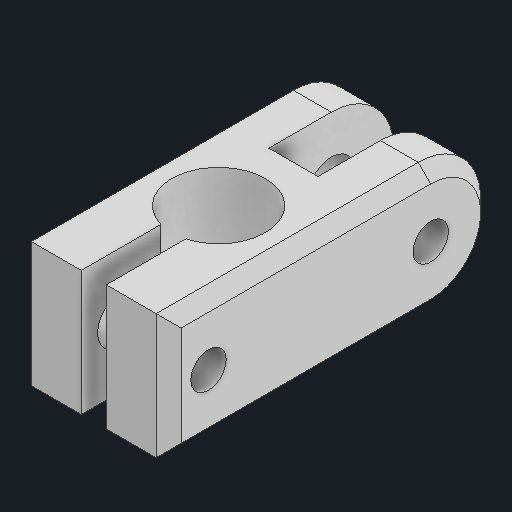
# Autodesk Inventor part: Part1
Saved by Autodesk Inventor 2025.1 (Build 291241020, 241B)
## iProperties
Created: 2025-05-01
Part Number: Part1
Material: Generic
Document SubType Name: Modeling
Designer: Joshua Eah
Density: 1 g/cm^3
Appearance: Default
Author: Joshua Eah
Autodesk Inventor part; units mm, degrees
ref_plane "YZ Plane" through (0, 0, 0) normal (1, 0, 0) x (0, 1, 0)
ref_plane "XZ Plane" through (0, 0, 0) normal (0, 1, 0) x (-1, 0, 0)
ref_plane "XY Plane" through (0, 0, 0) normal (0, 0, 1) x (1, 0, 0)
sketch "Sketch1" plane through (0, 0, 0) normal (0, 1, 0) x (-1, 0, 0)
  circle A0 centre (0, 0) radius 4.7625
  line L0 (7.62, -20.32) -> (-7.62, -20.32)
  line L1 (-7.62, -20.32) -> (-7.62, 12.7)
  line L2 (-7.62, 12.7) -> (7.62, 12.7)
  line L3 (7.62, 12.7) -> (7.62, -20.32)
  line L4 (1.27, 4.59) -> (1.27, 12.7)
  line L5 (-1.27, 4.59) -> (-1.27, 12.7)
  line L6 (0, 4.7625) -> (0, 12.7) construction
  dimension "d0" = 9.525
  dimension "d1" = 7.62
  dimension "d2" = 7.62
  dimension "d3" = 20.32
  dimension "d4" = 12.7
  dimension "d6" = 1.27
  dimension "d7" = 1.27
  constraints: 14 end point, 3 perpendicular, 3 point on circle, 2 parallel, 2 point on line, 1 centre point, 1 coincident, 1 horizontal, 1 midpoint
  measures "d0" diameter of A0
  measures "d1" distance from line of L3 A0.centre
  measures "d2" distance from line of L1 A0.centre
  measures "d3" distance from line of L0 A0.centre
  measures "d4" distance from line of L2 A0.centre
  measures "d6" distance between parallel lines of L4 L6
  measures "d7" distance between parallel lines of L5 L6
extrude "Extrusion1" add sketch "Sketch1" along normal blind 12.7 contours A0 L4 L2 L3 L0 L1 L5
sketch "Sketch2" plane through (-7.62, 0, -20.32) normal (-1, 0, 0) x (0, 0, 1)
  line L0 (0, 0) -> (33.02, 0) projected
  line L1 (33.02, 0) -> (33.02, 12.7) projected
  line L2 (0, 12.7) -> (33.02, 12.7) projected
  line L3 (0, 0) -> (0, 12.7) projected
  line L4 (0, 6.35) -> (33.02, 6.35) construction
  circle A0 centre (28.9687, 6.35) radius 1.75
  circle A1 centre (6.35, 6.35) radius 1.5
  point P0 (20.32, 0)
  dimension "d10" = 3.5
  dimension "d11" = 4.0513
  dimension "d20" = 3
  dimension "d21" = 6.35
  constraints: 2 centre point, 2 end point, 2 midpoint, 2 point on line
  measures "d10" diameter of A0
  measures "d11" distance from line of L1 A0.centre
  measures "d20" diameter of A1
  measures "d21" distance from line of A1.centre L3
hole "Hole1" at (-7.62, 6.35, 8.6487) at (-7.62, 6.35, -13.97) direction (1, 0, 0) diameter 3.6068 end through all clearance for "Flat Head Machine Screw" size "M3" standard "Ansi Metric M Profile"
fillet "Fillet1" radius 6.35 2 edges at (0, 12.7, -20.32) (0, 0, -20.32)
sketch "Sketch3" plane through (0, 12.7, 0) normal (0, 1, 0) x (1, 0, 0)
  line L0 (-7.62, 13.97) -> (7.62, 13.97) projected
  line L1 (-7.62, 13.97) -> (-7.62, -12.7) projected
  line L2 (-7.62, -12.7) -> (-1.27, -12.7) projected
  line L3 (-1.27, -12.7) -> (-1.27, -4.59) projected
  arc A0 (1.27, -4.59) -> (-1.27, -4.59) centre (0, 0) ccw projected
  line L4 (1.27, -4.59) -> (1.27, -12.7) projected
  line L5 (1.27, -12.7) -> (7.62, -12.7) projected
  line L6 (7.62, -12.7) -> (7.62, 13.97) projected
  line L7 (0, 4.7625) -> (0, 20.32) construction
  line L8 (7.62, 20.32) -> (-7.62, 20.32) projected
  line L9 (2.5, 4.0536) -> (2.5, 20.32)
  line L10 (-2.5, 4.0536) -> (-2.5, 20.32)
  line L11 (2.5, 7.62) -> (-2.5, 7.62)
  dimension "d22" = 2.5
  dimension "d23" = 2.5
  dimension "d26" = 12.7
  constraints: 8 end point, 4 point on line, 3 perpendicular, 3 point on circle, 1 midpoint
  measures "d22" distance between parallel lines of L7 L9
  measures "d23" distance between parallel lines of L10 L7
  measures "d26" distance from line of L7.end L11
extrude "Extrusion2" cut sketch "Sketch3" against normal through all contours L10 L8 L9 L0 | L0 L9 L11 L10
chamfer "Chamfer1" distance 1.27 angle 45 8 edges at (-7.62, 0, -0.6352) (-7.62, 10.8403, -18.4603) (-7.62, 12.7, -0.6352) (7.62, 12.7, -0.6353) (7.62, 10.8403, -18.4603) (7.62, 0, -0.6353) (-7.62, 6.35, 12.7) (7.62, 6.35, 12.7)
hole "Hole2" at (-7.62, 6.35, -13.97) at (-7.62, 6.35, 8.6487) direction (1, 0, 0) diameter 4.8006 depth 6.35 clearance for "Flat Head Machine Screw" size "M4" standard "Ansi Metric M Profile"
equation "\"d2\" = d1"
equation "\"d7\" = d6"
equation "\"d23\" = d22"
body "Solid1"
